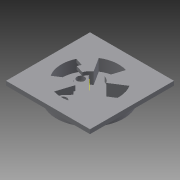
# Autodesk Inventor part: female 4 bay con
Saved by Autodesk Inventor 2015 (Build 190159000, 159)
## iProperties
Created: 2014-11-16
Part Number: female 4 bay con
Material: Generic
Document SubType Name: Modeling
Designer: ericd_000
Density: 1 g/cm^3
Appearance: Default
Author: ericd_000
Autodesk Inventor part; units mm, degrees
ref_plane "YZ Plane" through (0, 0, 0) normal (1, 0, 0) x (0, 1, 0)
ref_plane "XZ Plane" through (0, 0, 0) normal (0, 1, 0) x (-1, 0, 0)
ref_plane "XY Plane" through (0, 0, 0) normal (0, 0, 1) x (1, 0, 0)
sketch "Sketch5" plane through (0, 0, 0) normal (0, 0, 1) x (1, 0, 0)
  circle A0 centre (0, 0) radius 34
  dimension "d9" = 68
  constraints: 1 centre point, 1 coincident
  measures "d9" diameter of A0
extrude "Extrusion4" add sketch "Sketch5" along normal blind 5
sketch "Sketch6" plane through (0, 0, 5) normal (0, 0, 1) x (1, 0, 0)
  line L0 (0, 0) -> (-25.0441, 22.9955) construction
  circle A0 centre (0, 0) radius 34 construction
  line L1 (0, 0) -> (-18.239, 28.6939) construction
  line L2 (-25.0441, 22.9955) -> (-10.3123, 9.4687)
  line L3 (-18.239, 28.6939) -> (-7.5102, 11.8151)
  arc A1 (-7.5102, 11.8151) -> (-10.3123, 9.4687) centre (0, 0) ccw
  arc A2 (-18.239, 28.6939) -> (-25.0441, 22.9955) centre (0, 0) ccw
  dimension "d12" = 15
  dimension "d14" = 20
  constraints: 8 end point, 6 point on circle, 2 centre point, 2 concentric, 2 point on line
  measures "d12" angle of L0 L1
  measures "d14" distance of L0.end L2.end
extrude "Extrusion5" add sketch "Sketch6" along normal blind 14
sketch "Sketch7" plane through (-10.3123, 9.4687, 5) normal (-0.6763389, -0.7365906, 0) x (0.7365906, -0.6763389, 0)
  line L0 (-20, 14) -> (0, 14)
  line L1 (0, 14) -> (0, 8)
  line L2 (0, 8) -> (-20, 8)
  line L3 (-20, 8) -> (-20, 14)
  line L4 (14, -8.8) -> (14, 17.8) projected
  point P0 (14, -5)
  dimension "d17" = 6
  dimension "d18" = 20
  constraints: 8 end point, 2 parallel, 1 horizontal, 1 perpendicular
  measures "d17" distance between parallel lines of L0 L2
  measures "d18" distance of L0.start L0.end
revolve "Revolution1" add sketch "Sketch7" angle 25 about axis through (0, 0, 5) along (0, 0, 1)
sketch "Sketch8" plane through (0, 0, 5) normal (0, 0, 1) x (1, 0, 0)
  circle A0 centre (-21.5775, 10.5076) radius 4.5
  circle A1 centre (0, 0) radius 24 construction
  dimension "d25" = 48
  dimension "d21" = 9
  constraints: 1 centre point, 1 coincident, 3 other
  measures "d21" diameter of A0
extrude "Extrusion6" cut sketch "Sketch8" against normal up to surface (5 mm away)
pattern_circular "Circular Pattern1" count 4 over 360 about axis through (0, 0, 5) along (0, 0, 1) of "Extrusion6", "Revolution1", "Extrusion5"
sketch "Sketch9" plane through (0, 0, 0) normal (0, 0, -1) x (-1, 0, 0)
  circle A0 centre (0, 0) radius 34
  circle A1 centre (0, 0) radius 40
  dimension "d31" = 68
  dimension "d32" = 6
  constraints: 2 centre point, 2 coincident
  measures "d31" diameter of A0
  measures "d32" radial gap between concentric circles of A1 A0
extrude "Extrusion7" add sketch "Sketch9" against normal blind 19
sketch "Sketch10" plane through (0, 0, 19) normal (0, 0, 1) x (1, 0, 0)
  circle A0 centre (0, 0) radius 40
  line L0 (-50, 50) -> (50, 50)
  line L1 (50, 50) -> (50, -50)
  line L2 (50, -50) -> (-50, -50)
  line L3 (-50, -50) -> (-50, 50)
  point P0 (-50, 0)
  point P1 (0, 50)
  dimension "d35" = 100
  dimension "d36" = 100
  dimension "d37" = 80
  constraints: 8 end point, 2 midpoint, 2 parallel, 1 centre point, 1 coincident, 1 horizontal, 1 horizontal alignment, 1 perpendicular, 1 vertical alignment
  measures "d35" distance of L0.start L0.end
  measures "d36" distance of L2.end L0.start
  measures "d37" diameter of A0
extrude "Extrusion8" add sketch "Sketch10" against normal blind 5
sketch "Sketch11" plane through (0, 0, 19) normal (0, 0, 1) x (1, 0, 0)
  line L0 (-7.5102, 11.8151) -> (-18.239, 28.6939) projected
  line L1 (-13.3478, 4.2234) -> (-32.416, 10.2569) projected
  arc A0 (-12.8746, 20.2545) -> (-22.8819, 7.2402) centre (0, 0) ccw
  arc A1 (-32.416, 10.2569) -> (-28.6939, -18.239) centre (0, 0) ccw projected
  arc A2 (-18.239, 28.6939) -> (-32.416, 10.2569) centre (0, 0) ccw
  line L2 (-30.7733, 14.4571) -> (-21.1185, 11.4021)
  dimension "d40" = 10
  dimension "d41" = 4.5
  constraints: 6 point on circle, 2 centre point, 2 concentric, 2 end point, 2 midpoint, 1 parallel
  measures "d40" distance of L1.end A0.end
  measures "d41" distance between parallel lines of L1 L2
extrude "Extrusion9" cut sketch "Sketch11" against normal up to surface (6 mm away) contours A0 L1 A2 L2
sketch "Sketch14" plane through (0, 0, 13) normal (0, 0, -1) x (-0.865517, 0.5008796, 0)
  line L0 (33.1941, 7.3589) -> (13.6681, 3.0302)
  line L1 (13.6681, 3.0302) -> (13.6681, -3.0302)
  line L2 (13.6681, -3.0302) -> (23.4311, -5.1946)
  line L3 (23.4311, -5.1946) -> (13.6681, -3.0302) projected
  line L4 (23.4311, -5.1946) -> (33.876, -2.9009)
  line L5 (33.876, -2.9009) -> (33.1941, 7.3589)
  point P0 (0, 0)
  constraints: 10 end point, 1 collinear, 1 vertical
extrude "Extrusion10" cut sketch "Sketch14" against normal blind 10
sketch "Sketch15" plane through (-10.3123, 9.4687, 5) normal (-0.6763389, -0.7365906, 0) x (0.7365906, -0.6763389, 0)
  line L0 (0, 0) -> (0, 14) projected
  line L1 (-20, 14) -> (0, 14)
  line L2 (0, 14) -> (0, 10)
  line L3 (0, 10) -> (-20, 10)
  line L4 (-20, 10) -> (-20, 14)
  line L5 (14, -8.8) -> (14, 17.8) projected
  point P0 (14, -5)
  dimension "d48" = 4
  constraints: 8 end point, 2 parallel, 1 horizontal, 1 perpendicular, 1 point on line
  measures "d48" distance between parallel lines of L1 L3
revolve "Revolution2" add sketch "Sketch15" angle 25 about axis through (0, 0, 5) along (0, 0, 1)
sketch "Sketch16" plane through (0, 0, 19) normal (0, 0, 1) x (1, 0, 0)
  line L0 (-32.416, 10.2569) -> (-23.0004, 7.2777)
  line L1 (-13.3478, 4.2234) -> (-32.416, 10.2569) projected
  line L2 (-21.2392, 11.4403) -> (-30.7733, 14.4571)
  arc A0 (-30.7733, 14.4571) -> (-32.416, 10.2569) centre (0, 0) ccw
  arc A1 (-21.2392, 11.4403) -> (-23.0004, 7.2777) centre (0, 0) ccw
  arc A2 (-32.416, 10.2569) -> (-28.6939, -18.239) centre (0, 0) ccw projected
  dimension "d50" = 4.5
  dimension "d51" = 10
  constraints: 4 end point, 4 point on circle, 2 centre point, 2 concentric, 1 parallel, 1 point on line
  measures "d50" distance between parallel lines of L2 L0
  measures "d51" distance of L2.start L2.end
extrude "Extrusion11" cut sketch "Sketch16" against normal blind 10
body "Solid2"
